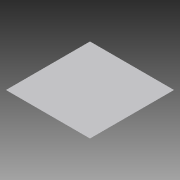
# Autodesk Inventor part: Ground
Saved by Autodesk Inventor 2013 (Build 170138000, 138)
## iProperties
Created: 2013-01-29
Part Number: Ground
Material: Carpet
Document SubType Name: Sheet Metal
Designer: carneeki
Density: 1 g/cm^3
Sheet Metal Rule: Default
Author: carneeki
Autodesk Inventor part; units mm, degrees
ref_plane "YZ Plane" through (0, 0, 0) normal (1, 0, 0) x (0, 1, 0)
ref_plane "XZ Plane" through (0, 0, 0) normal (0, 1, 0) x (-1, 0, 0)
ref_plane "XY Plane" through (0, 0, 0) normal (0, 0, 1) x (1, 0, 0)
sketch "Sketch1" plane through (0, 0, 0) normal (0, 1, 0) x (-1, 0, 0)
  line L0 (0, 0) -> (1219.2, 0)
  line L1 (1219.2, 0) -> (1422.4, 351.9527)
  line L2 (1422.4, 351.9527) -> (812.8, 1407.8109)
  line L3 (812.8, 1407.8109) -> (406.4, 1407.8109)
  line L4 (406.4, 1407.8109) -> (-203.2, 351.9527)
  line L5 (-203.2, 351.9527) -> (0, 0)
  dimension "d7" = 1219.2
  dimension "d8" = 406.4
  dimension "d9" = 120
  dimension "d10" = 1219.2
  dimension "d11" = 120
  dimension "d12" = 406.4
  dimension "d13" = 1219.2
  dimension "d14" = 120
  measures "d7" distance of L0.start L0.end
  measures "d8" distance of L0.end L1.end
  measures "d9" angle of L1 L0
  measures "d10" distance of L1.end L2.end
  measures "d11" angle of L2 L1
  measures "d12" distance of L2.end L3.end
  measures "d13" distance of L3.end L4.end
  measures "d14" angle of L4 L3
extrude "Plate1" add sketch "Sketch1" along normal blind 3.048
equation "\"BendRadius\" = Thickness"
equation "\"BendReliefWidth\" = Thickness"
equation "\"BendReliefDepth\" = 0.5 * Thickness"
equation "\"CornerReliefSize\" = 4 * Thickness"
equation "\"MinimumRemnant\" = 2 * Thickness"
equation "\"TransitionRadius\" = BendRadius"
equation "\"JacobiRadiusSize\" = BendRadius"
equation "\"GapSize\" = Thickness"
equation "\"d2\" = BendRadius"
equation "\"Thickness\" = 3.048"
body "Solid1"
